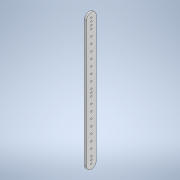
# Autodesk Inventor part: Intake Mounting Bracket
Saved by Autodesk Inventor 2022 (Build 260153000, 153)
## iProperties
Created: 2022-09-30
Part Number: Intake Mounting Bracket
Material: Generic
Document SubType Name: Modeling
Designer: matt
Density: 1 g/cm^3
Appearance: Default
Author: matt
Autodesk Inventor part; units mm, degrees
ref_plane "YZ Plane" through (0, 0, 0) normal (1, 0, 0) x (0, 1, 0)
ref_plane "XZ Plane" through (0, 0, 0) normal (0, 1, 0) x (-1, 0, 0)
ref_plane "XY Plane" through (0, 0, 0) normal (0, 0, 1) x (1, 0, 0)
sketch "Sketch1" plane through (0, 0, 0) normal (1, 0, 0) x (0, 1, 0)
  circle A0 centre (144, 0) radius 2
  arc A1 (288, 0) -> (288, 0) centre (288, 0) ccw
  circle A2 centre (288, 0) radius 2
  circle A3 centre (0, 0) radius 2
  line L0 (0, 0) -> (288, 0) construction
  line L1 (0, 0) -> (288, 0) construction
  line L2 (0, -12) -> (312, -12)
  line L3 (312, 12) -> (0, 12)
  arc A4 (0, 12) -> (0, -12) centre (0, 0) ccw
  circle A5 centre (9.7, 100) radius 1.6
  circle A6 centre (9.7, 108) radius 4.5
  circle A7 centre (9.7, 116) radius 1.6
  circle A8 centre (9.7, 124) radius 4.5
  circle A9 centre (144, 0) radius 4.5
  circle A10 centre (8, 0) radius 4.35
  circle A11 centre (16, 0) radius 2
  circle A12 centre (24, 0) radius 4.35
  circle A13 centre (32, 0) radius 2
  circle A14 centre (40, 0) radius 4.35
  circle A15 centre (48, 0) radius 2
  circle A16 centre (56, 0) radius 4.35
  circle A17 centre (64, 0) radius 2
  circle A18 centre (72, 0) radius 4.35
  circle A19 centre (80, 0) radius 2
  circle A20 centre (88, 0) radius 4.35
  circle A21 centre (96, 0) radius 2
  circle A22 centre (104, 0) radius 4.35
  circle A23 centre (112, 0) radius 2
  circle A24 centre (120, 0) radius 4.35
  circle A25 centre (128, 0) radius 2
  circle A26 centre (136, 0) radius 4.35
  circle A27 centre (144, 0) radius 2
  circle A28 centre (152, 0) radius 4.35
  circle A29 centre (160, 0) radius 2
  circle A30 centre (168, 0) radius 4.35
  circle A31 centre (176, 0) radius 2
  circle A32 centre (184, 0) radius 4.35
  circle A33 centre (192, 0) radius 2
  circle A34 centre (200, 0) radius 4.35
  circle A35 centre (208, 0) radius 2
  circle A36 centre (216, 0) radius 4.35
  circle A37 centre (224, 0) radius 2
  circle A38 centre (232, 0) radius 4.35
  circle A39 centre (240, 0) radius 2
  circle A40 centre (248, 0) radius 4.35
  circle A41 centre (256, 0) radius 2
  circle A42 centre (264, 0) radius 4.35
  circle A43 centre (272, 0) radius 2
  circle A44 centre (280, 0) radius 4.35
  circle A45 centre (288, 0) radius 2
  circle A46 centre (296, 0) radius 4.35
  circle A47 centre (296, 0) radius 2
  circle A48 centre (304, 0) radius 2
  circle A49 centre (312, 0) radius 2
  arc A50 (312, -12) -> (312, 12) centre (312, 0) ccw
  circle A51 centre (8, 0) radius 2
  circle A52 centre (152, 0) radius 2
  point P0 (148.082969, -1.891921)
  point P1 (139.917031, -1.891921)
  point P2 (139.917031, 1.891921)
  point P3 (148.082969, 1.891921)
  dimension "d0" = 4
  dimension "d1" = 4
  dimension "d2" = 144
  dimension "d3" = 4
  dimension "d4" = 144
  dimension "d6" = 3.2
  dimension "d7" = 9
  dimension "d8" = 8
  dimension "d9" = 8
  dimension "d10" = 8
  dimension "d11" = 9
  dimension "d12" = 8.7
  dimension "d13" = 8
  dimension "d16" = 16
  dimension "d27" = 8
  dimension "d32" = 24
  dimension "d33" = 4
  dimension "d34" = 4
  constraints: 53 centre point, 10 end point, 7 coincident, 4 point on circle, 3 horizontal, 2 coincident with centre, 2 equal length, 2 equal radius, 2 midpoint, 2 tangent, 1 point on line, 78 other
  measures "d0" diameter of A2
  measures "d1" diameter of A0
  measures "d2" distance of A1.centre A0.centre
  measures "d3" diameter of A3
  measures "d4" distance of L0.start A0.centre
  measures "d6" diameter of A5
  measures "d7" diameter of A6
  measures "d8" distance of A6.centre A5.centre
  measures "d9" distance of A7.centre A6.centre
  measures "d10" distance of A8.centre A7.centre
  measures "d11" diameter of A9
  measures "d12" diameter of A10
  measures "d13" distance of L0.start A10.centre
  measures "d16" distance of L0.start A11.centre
  measures "d27" distance of L1.end A47.centre
  measures "d32" diameter of A50
  measures "d33" diameter of A51
  measures "d34" diameter of A52
sketch "Sketch1 outline for Extrusion1" plane through (0, 0, 0) normal (1, 0, 0) x (0, 1, 0)
  line L0 (0, -12) -> (312, -12)
  arc A0 (312, -12) -> (312, 12) centre (312, 0) ccw
  line L1 (312, 12) -> (0, 12)
  arc A1 (0, 12) -> (0, -12) centre (0, 0) ccw
  circle A2 centre (0, 0) radius 2
  circle A3 centre (16, 0) radius 2
  circle A4 centre (32, 0) radius 2
  circle A5 centre (48, 0) radius 2
  circle A6 centre (64, 0) radius 2
  circle A7 centre (80, 0) radius 2
  circle A8 centre (96, 0) radius 2
  circle A9 centre (112, 0) radius 2
  circle A10 centre (128, 0) radius 2
  circle A11 centre (160, 0) radius 2
  circle A12 centre (176, 0) radius 2
  circle A13 centre (192, 0) radius 2
  circle A14 centre (208, 0) radius 2
  circle A15 centre (224, 0) radius 2
  circle A16 centre (240, 0) radius 2
  circle A17 centre (256, 0) radius 2
  circle A18 centre (272, 0) radius 2
  circle A19 centre (288, 0) radius 2
  circle A20 centre (296, 0) radius 2
  circle A21 centre (304, 0) radius 2
  circle A22 centre (312, 0) radius 2
  circle A23 centre (8, 0) radius 2
  circle A24 centre (152, 0) radius 2
  circle A25 centre (144, 0) radius 2
extrude "Extrusion1" add sketch "Sketch1 outline for Extrusion1" along normal blind 4.7625
sketch "Sketch1 outline for Extrusion2" plane through (0, 0, 0) normal (1, 0, 0) x (0, 1, 0)
  circle A0 centre (24, 0) radius 4.35
  circle A1 centre (56, 0) radius 4.35
  circle A2 centre (88, 0) radius 4.35
  circle A3 centre (120, 0) radius 4.35
  circle A4 centre (184, 0) radius 4.35
  circle A5 centre (216, 0) radius 4.35
  circle A6 centre (248, 0) radius 4.35
  circle A7 centre (280, 0) radius 4.35
extrude "Extrusion2" add sketch "Sketch1 outline for Extrusion2" against normal blind 1.651 from surface at 0
equation "\"d4\" = d2"
body "Solid1"
